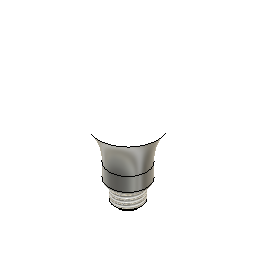
Day9LightBulb (Autodesk Fusion 360 design; units mm, degrees)
part number: 2025-11-26-19-18-02-019
Autodesk Fusion 360 part; units mm, degrees
sketch "Sketch1" plane through (0, 0, 0) normal (0, 0, 1) x (1, 0, 0)
  circle A0 centre (0, 0) radius 15
  dimension "d1" = 30
  constraint coincident A0.centre origin
  measures "d1" diameter of A0
extrude "Extrude2" add sketch "Sketch1" along normal blind 40
sketch "Sketch2" plane through (0, 0, 0) normal (0, 1, 0) x (1, 0, 0)
  line L0 (-15, -40) -> (15, -40)
  line L1 (0, -40) -> (0, -60)
  point P0 (-15, -40)
  point P1 (-15, -40)
  point P2 (15, -40)
  dimension "d6" = 20
  constraint coincident P1 P0
  constraint coincident P2 L0.end
  constraint midpoint L0 L1.start
  constraint perpendicular L0 L1
  measures "d6" distance of L1.start L1.end
sphere "SpherePrimitive1" add diameter 61 placed x (1, 0, 0) y (0, 0, -1) z (0, 1, 0) at (0, 0, 60)
fillet "Fillet1" radius 45 1 edges at (-13.9849, 5.4242, 33.4435)
fillet "Fillet2" radius 3 1 edges at (-13.9849, -5.4242, 0)
cylinder "CylinderPrimitive1" add diameter 22 height 15 placed x (0, 1, 0) y (1, 0, 0) z (0, 0, -1) at (0, 0, 0)
thread "Thread1" "ISO Metric profile 22.0 M22x3 M22x3 6g" major diameter 21.7645 minor diameter 18.3374 pitch 3 angle 60 resizes the face on face at (-1.0952, 10.9453, -5)
chamfer "Chamfer1" distance 3 angle 45 1 edges at (-3.9352, -10.1458, -15) measured on face at (-0.3528, 2.3404, -15)
